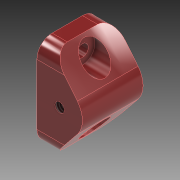
# Autodesk Inventor part: F4C9-200-002 Side Bearing Block
Saved by Autodesk Inventor 2021 (Build 250183000, 183)
## iProperties
ItemSpecifications: {"_id":"606db26a1848470009a25198","finish":"543ef1f380da5b0c476373c1","finish_location":null,"material":"5515e170db035c20ce34af9a","process_initialism":null,"quotes":null,"current_quote":null,"quantity_ordered":20,"features":null,"hardware":null,"threading":null,"part_markings":[],"surface_roughness":null,"tolerance":null,"weld_quantity":null,"Notes":"","certifications":[],"part":null,"revision_num":0,"last_history":null,"inspection_requirement_details":{"inspection_requirement":"std","customer_data_sheet":null},"feedback":null}
Created: 2020-08-09
Part Number: F4C9-200-002 Side Bearing Block
Material: Aluminum 6061
Document SubType Name: Modeling
Designer: Cal
Density: 2.7 g/cm^3
Appearance: Reflective - Red
Author: Cal
Autodesk Inventor part; units mm, degrees
ref_plane "YZ Plane" through (0, 0, 0) normal (1, 0, 0) x (0, 1, 0)
ref_plane "XZ Plane" through (0, 0, 0) normal (0, 1, 0) x (-1, 0, 0)
sketch "Sketch1" plane through (0, 0, 0) normal (0, 0, 1) x (1, 0, 0)
  circle A0 centre (0, 0) radius 9.525 construction
  circle A1 centre (0, 0) radius 1.9812
  line L0 (-9.525, 19.05) -> (-9.525, -19.05)
  line L1 (-9.525, 19.05) -> (-3.175, 19.05)
  line L2 (-3.175, 19.05) -> (7.4009, 5.996)
  line L3 (-9.525, -19.05) -> (-3.175, -19.05)
  line L4 (-3.175, -19.05) -> (7.4009, -5.996)
  arc A2 (7.4009, -5.996) -> (7.4009, 5.996) centre (0, 0) ccw
  point P0 (-9.525, 0)
  dimension "d0" = 19.05
  dimension "d1" = 3.9624
  dimension "d3" = 38.1
  dimension "d17" = 6.35
  dimension "d26" = 9.525
  constraints: 10 end point, 3 centre point, 3 coincident, 3 tangent, 2 horizontal, 2 midpoint, 2 point on circle, 1 horizontal alignment, 1 vertical, 1 vertical alignment
  measures "d0" diameter of A0
  measures "d1" diameter of A1
  measures "d3" distance of L0.start L0.end
  measures "d17" distance of L0.start L1.end
  measures "d26" radius of A2
extrude "Extrusion1" add sketch "Sketch1" along normal mid plane 25.4
sketch "Sketch2" plane through (-9.525, -19.05, 12.7) normal (-1, 0, 0) x (0, 0, 1)
  circle A0 centre (-12.7, 19.05) radius 2.4892 construction
  line L0 (-25.4, 0) -> (-25.4, 38.1) projected
  circle A1 centre (-12.7, 31.75) radius 2.4892
  circle A2 centre (-12.7, 6.35) radius 2.4892
  circle A3 centre (-12.7, 19.05) radius 2.4892 construction
  dimension "d6" = 4.9784
  dimension "d9" = 12.7
  dimension "d12" = 12.7
  constraints: 4 centre point, 2 vertical, 1 coincident, 6 other
  measures "d6" diameter of A0
  measures "d9" distance of A0.centre A1.centre
  measures "d12" distance of A0.centre A2.centre
extrude "Extrusion2" cut sketch "Sketch2" against normal through all
ref_plane "Work Plane1" through (-3.175, -19.05, 12.7) normal (-1, 0, 0) x (0, 0, 1)
sketch "Sketch3" plane through (-3.175, -19.05, 12.7) normal (-1, 0, 0) x (0, 0, 1)
  circle A0 centre (-12.7, 31.75) radius 2.4892 projected
  circle A1 centre (-12.7, 6.35) radius 2.4892 projected
  circle A2 centre (-12.7, 31.75) radius 5.2705
  circle A3 centre (-12.7, 6.35) radius 5.2705
  point P0 (-12.7, 19.05)
  dimension "d18" = 10.541
  dimension "d19" = 10.541
  constraints: 2 centre point, 2 coincident
  measures "d18" diameter of A2
  measures "d19" diameter of A3
extrude "Extrusion3" cut sketch "Sketch3" against normal through all
thread "Thread1" size "10-24 UNC" class "2B" standard "ANSI Unified Screw Threads" length 25.4
fillet "Fillet1" radius 6.35 4 edges at (-6.35, 19.05, 12.7) (-6.35, 19.05, -12.7) (-6.35, -19.05, 12.7) (-6.35, -19.05, -12.7)
sketch "Sketch5" plane through (0, 0, -12.7) normal (0, 0, -1) x (-1, 0, 0)
  circle A0 centre (0, 0) radius 1.9812 projected
extrude "Extrusion5" [suppressed]
equation "\"d19\" = d18"
body "Solid1"
